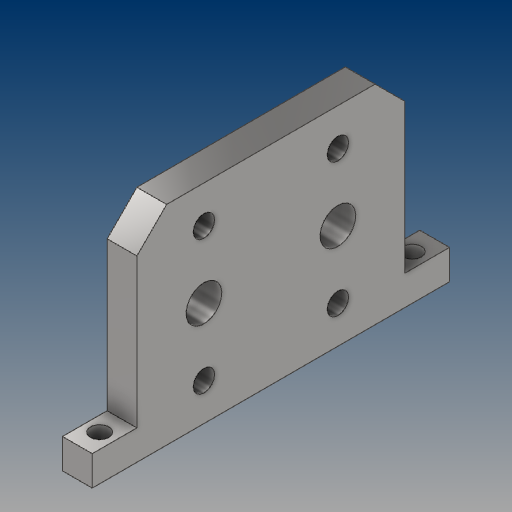
# Autodesk Inventor part: 22_Hop_so_ngang
Saved by Autodesk Inventor 2021 (Build 250183000, 183)
## iProperties
Created: 2024-04-07
Part Number: 22_Hop_so_ngang
Material: Stainless Steel, Austenitic
Document SubType Name: Modeling
Designer: Admin
Density: 8 g/cm^3
Appearance: Semi-Polished
Author: Admin
Autodesk Inventor part; units mm, degrees
ref_plane "YZ Plane" through (0, 0, 0) normal (1, 0, 0) x (0, 1, 0)
ref_plane "XZ Plane" through (0, 0, 0) normal (0, 1, 0) x (-1, 0, 0)
ref_plane "XY Plane" through (0, 0, 0) normal (0, 0, 1) x (1, 0, 0)
sketch "Sketch1" plane through (0, 0, 0) normal (1, 0, 0) x (0, 1, 0)
  line L0 (-35, 60) -> (35, 60)
  line L1 (35, 60) -> (35, -60)
  line L2 (35, -60) -> (-35, -60)
  line L3 (-35, -60) -> (-35, 60)
  line L4 (-35, 60) -> (35, -60) construction
  line L5 (35, 60) -> (-35, -60) construction
  line L6 (0, 60) -> (0, -60) construction
  line L7 (20, 60) -> (35, -15)
  line L8 (0, 22.5) -> (0, -22.5)
  line L9 (-35, 0) -> (35, 0) construction
  circle A0 centre (0, 22.5) radius 18 construction
  circle A1 centre (0, -22.5) radius 26 construction
  line L10 (-35, 51) -> (35, 51)
  circle A2 centre (0, 22.5) radius 6
  circle A3 centre (0, -22.5) radius 6
  point P0 (0, 0)
  point P1 (21.8, 51)
  dimension "d0" = 35
  dimension "d1" = 120
  dimension "d2" = 45
  dimension "d3" = 52
  dimension "d4" = 36
  dimension "d5" = 75
  dimension "d6" = 15
  dimension "d7" = 9
  dimension "d8" = 12
  dimension "d9" = 12
  constraints: 22 end point, 6 midpoint, 6 point on line, 4 centre point, 4 coincident, 2 parallel, 2 perpendicular, 1 horizontal, 1 symmetric about line
  measures "d0" distance between parallel lines of L1 L6
  measures "d1" distance between parallel lines of L0 L2
  measures "d2" distance of L8.start L8.end
  measures "d3" diameter of A1
  measures "d4" diameter of A0
  measures "d5" distance from line of L0 L7.end
  measures "d6" distance from line of L1 L7.start
  measures "d7" distance between parallel lines of L0 L10
  measures "d8" diameter of A3
  measures "d9" diameter of A2
extrude "Extrusion1" add sketch "Sketch1" along normal blind 10
sketch "Sketch2" plane through (0, 35, -15) normal (0, 1, 0) x (1, 0, 0)
  line L0 (0, 45) -> (0, -75) construction
  line L1 (10, 45) -> (10, -75) projected
  line L2 (0, 45) -> (10, 45) projected
  line L3 (0, 0) -> (0, -66) projected
  line L4 (0, -66) -> (10, -66) construction
  line L5 (10, 0) -> (10, -66) projected
  line L6 (0, 0) -> (10, 0) projected
  line L7 (0, 45) -> (10, 45) projected
  line L8 (0, 45) -> (10, 45)
  line L9 (10, 45) -> (10, 30)
  line L10 (10, 30) -> (0, 30)
  line L11 (0, 30) -> (0, 45)
  line L12 (0, -75) -> (10, -75) projected
  line L13 (0, 45) -> (0, -75) projected
  line L14 (0, -75) -> (10, -75)
  line L15 (10, -75) -> (10, -60)
  line L16 (10, -60) -> (0, -60)
  line L17 (0, -60) -> (0, -75)
  point P0 (0, -15)
  point P1 (0, 30)
  point P2 (0, -60)
  dimension "d36" = 15
  dimension "d37" = 15
  constraints: 16 end point, 4 parallel, 2 horizontal, 2 perpendicular, 2 point on line
  measures "d36" distance between parallel lines of L12 L16
  measures "d37" distance between parallel lines of L2 L10
extrude "Extrusion2" cut sketch "Sketch2" against normal blind 60 contours L1 L10 L11 L2 | L1 L12 L13 L3 L16
sketch "Sketch3" plane through (10, 0, 0) normal (1, 0, 0) x (0, 0, -1)
  line L0 (45, 35) -> (-45, 35) projected
  line L1 (-60, -35) -> (60, -35) projected
  line L2 (60, -35) -> (60, -25) projected
  circle A0 centre (-22.5, 0) radius 6 projected
  circle A1 centre (22.5, 0) radius 6 projected
  line L3 (-22.5, 22.5) -> (-22.5, -22.5)
  line L4 (-22.5, 0) -> (22.5, 0) construction
  line L5 (22.5, 22.5) -> (22.5, -22.5)
  line L6 (-60, -25) -> (-60, -35) projected
  line L7 (45, -25) -> (45, 35) projected
  line L8 (-45, 35) -> (-45, -25) projected
  line L9 (-45, -25) -> (-60, -25) projected
  line L10 (60, -25) -> (45, -25) projected
  point P0 (0, 0)
  dimension "d16" = 45
  constraints: 6 end point, 2 midpoint, 2 symmetric about line, 2 vertical, 1 horizontal, 1 parallel
  measures "d16" distance of L5.start L5.end
hole "Hole1" at (10, 22.5, 22.5) at (10, -22.5, 22.5) at (10, 22.5, -22.5) at (10, -22.5, -22.5) direction (-1, 0, 0) diameter 7.2 end through all
sketch "Sketch4" plane through (0, -25, -15) normal (0, 1, 0) x (1, 0, 0)
  line L0 (0, 30) -> (0, 45) projected
  line L1 (10, -60) -> (10, -75) projected
  line L2 (10, 45) -> (10, 30) projected
  line L3 (0, 45) -> (10, 45) projected
  line L4 (0, 30) -> (0, 45) projected
  line L5 (10, 30) -> (0, 30) projected
  line L6 (5, -75) -> (5, 45)
  line L7 (10, 45) -> (10, 30) projected
  line L8 (0, 45) -> (10, 45) projected
  line L9 (10, 30) -> (0, 30) projected
  line L10 (0, -75) -> (0, -60) projected
  line L11 (10, -75) -> (0, -75) projected
  line L12 (0, -60) -> (10, -60) projected
  point P0 (0, -15)
  point P1 (5, -67.5)
  point P2 (5, 37.5)
  dimension "d24" = 7.5
  dimension "d38" = 7.5
  constraints: 2 end point, 2 midpoint, 2 point on line
  measures "d24" distance from line of L3 point (5, 37.5)
  measures "d38" distance of L6.start point (5, -67.5)
hole "Hole2" at (5, -25, 52.5) at (5, -25, -52.5) direction (0, -1, 0) diameter 6.2 end through all
chamfer "Chamfer1" distance 10 angle 45 2 edges at (5, 35, -45) (5, 35, 45)
body "Solid1"
